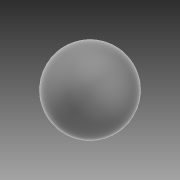
# Autodesk Inventor part: FRC 2016 Ball
Saved by Autodesk Inventor 2021 (Build 250183000, 183)
## iProperties
Created: 2021-02-26
Part Number: FRC 2016 Ball
Material: Generic
Document SubType Name: Modeling
Surface Area: 1641.73 cm^2
Volume: 6255 cm^3
Appearance: Smooth - Dark Gray
Autodesk Inventor part; units mm, degrees
ref_plane "YZ Plane" through (0, 0, 0) normal (1, 0, 0) x (0, 1, 0)
ref_plane "XZ Plane" through (0, 0, 0) normal (0, 1, 0) x (-1, 0, 0)
ref_plane "XY Plane" through (0, 0, 0) normal (0, 0, 1) x (1, 0, 0)
sketch "Sketch1" plane through (0, 0, 0) normal (0, 0, 1) x (1, 0, 0)
  arc A0 (0, -114.3) -> (0, 114.3) centre (0, 0) ccw
  line L0 (0, 114.3) -> (0, -114.3)
  point P0 (0, 0)
  dimension "d0" = 228.6
  constraints: 2 end point, 2 point on circle, 2 vertical alignment, 1 centre point, 1 coincident, 1 midpoint, 1 vertical
  measures "d0" diameter of A0
revolve "Revolution1" add sketch "Sketch1" angle 360 about axis through (0, 114.3, 0) along (0, -1, 0)
body "Solid1"
